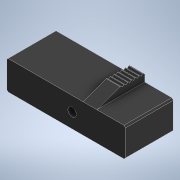
# Autodesk Inventor part: Magazin2_Stössel
Saved by Autodesk Inventor 2021 (Build 250183000, 183)
## iProperties
Created: 2024-08-28
Part Number: Magazin2_Stössel
Material: Generic
Document SubType Name: Modeling
Designer: Lukas
Density: 1 g/cm^3
Appearance: Default
Author: Lukas
Autodesk Inventor part; units mm, degrees
ref_plane "YZ Plane" through (0, 0, 0) normal (1, 0, 0) x (0, 1, 0)
ref_plane "XZ Plane" through (0, 0, 0) normal (0, 1, 0) x (-1, 0, 0)
ref_plane "XY Plane" through (0, 0, 0) normal (0, 0, 1) x (1, 0, 0)
sketch "Sketch1" plane through (0, 0, 0) normal (0, 0, 1) x (1, 0, 0)
  line L0 (-19.85, 4.85) -> (19.85, 4.85)
  line L1 (19.85, 4.85) -> (19.85, -4.85)
  line L2 (19.85, -4.85) -> (-19.85, -4.85)
  line L3 (-19.85, -4.85) -> (-19.85, 4.85)
  line L4 (5.7, 4.85) -> (5.7, 7.65)
  line L5 (5.7, 7.65) -> (10.3, 7.65)
  line L6 (10.3, 7.65) -> (10.3, 4.85)
  point P0 (0, 0)
  point P1 (0, 4.85)
  point P2 (-19.85, 0)
  point P3 (8, 7.65)
  dimension "d0" = 9.7
  dimension "d1" = 39.7
  dimension "d2" = 4.6
  dimension "d3" = 2.8
  dimension "d28" = 8
  constraints: 14 end point, 3 midpoint, 3 perpendicular, 2 parallel, 2 point on line, 1 horizontal, 1 horizontal alignment, 1 vertical, 1 vertical alignment
  measures "d0" distance of L2.end L0.start
  measures "d1" distance of L0.start L0.end
  measures "d2" distance of L4.end L5.end
  measures "d3" distance of L5.end L6.end
  measures "d28" horizontal distance of point (8, 7.65) point (0, 4.85)
extrude "Extrusion1" add sketch "Sketch1" along normal blind 16
sketch "Sketch2" plane through (10.3, 4.85, 0) normal (1, 0, 0) x (0, 0, -1)
  line L0 (0, 0) -> (0, 2.8) projected
  line L1 (0, 2.8) -> (-16, 2.8) projected
  line L2 (-16, 0) -> (-16, 2.8) projected
  line L3 (0, 0) -> (-16, 0) projected
  line L4 (0, 0) -> (-16, 0) projected
  line L5 (-16, 0) -> (-8.25, 2.8)
  line L6 (0, 2.8) -> (-16, 2.8) projected
  line L7 (-6.75, 2.8) -> (-6.25, 2.3)
  line L8 (-6.25, 2.3) -> (-5.75, 2.8)
  line L9 (-4.25, 2.8) -> (-3.75, 2.3)
  line L10 (-3.75, 2.3) -> (-3.25, 2.8)
  line L11 (-1.75, 2.8) -> (-1.25, 2.3)
  line L12 (-1.25, 2.3) -> (-0.75, 2.8)
  line L13 (0, 2.8) -> (-16, 2.8) projected
  line L14 (-3, 2.8) -> (-2.5, 2.3)
  line L15 (-2.5, 2.3) -> (-2, 2.8)
  line L16 (-5.5, 2.8) -> (-5, 2.3)
  line L17 (-5, 2.3) -> (-4.5, 2.8)
  line L18 (-7, 2.8) -> (-7.5, 2.3)
  line L19 (-7.5, 2.3) -> (-8, 2.8)
  line L20 (-0.5, 2.8) -> (0, 2.3)
  line L21 (0, 0) -> (0, 2.8) projected
  point P0 (0, -4.85)
  dimension "d8" = 0.75
  dimension "d9" = 1
  dimension "d13" = 0.25
  dimension "d14" = 0.25
  dimension "d15" = 0.25
  dimension "d16" = 0.25
  dimension "d17" = 0.25
  dimension "d18" = 0.25
  dimension "d26" = 0.5
  constraints: 28 end point, 14 perpendicular, 4 point on line, 2 horizontal alignment, 2 parallel, 14 other
  measures "d8" distance from line of L0 L12.end
  measures "d9" distance of L11.start L12.end
  measures "d13" distance of L11.start L15.end
  measures "d14" distance of L10.end L14.start
  measures "d15" distance of L17.end L9.start
  measures "d16" distance of L8.end L16.start
  measures "d17" distance of L7.start L18.start
  measures "d18" distance of L5.end L19.end
  measures "d26" distance of L0.end L20.start
extrude "Extrusion2" cut sketch "Sketch2" against normal through all contours L20 L1 L0 | L2 L1 L5 | L12 L11 L1 | L1 L18 L19 | L15 L14 L1 | L1 L8 L7 | L10 L9 L1 | L1 L17 L16
sketch "Sketch3" plane through (0, 0, 16) normal (0, 0, 1) x (1, 0, 0)
  circle A0 centre (2, 0) radius 1.4
  point P0 (0, 0)
  dimension "d19" = 2
  dimension "d20" = 2.8
  constraints: 1 centre point, 1 horizontal alignment
  measures "d19" distance of point (0, 0) A0.centre
  measures "d20" diameter of A0
extrude "Extrusion3" cut sketch "Sketch3" against normal blind 10
chamfer "Chamfer1" distance 0.5 angle 45 4 edges at (-19.85, -4.85, 8) (-19.85, 4.85, 8) (19.85, -4.85, 8) (19.85, 4.85, 8)
equation "\"d14\" = d13"
equation "\"d15\" = d14"
equation "\"d16\" = d15"
equation "\"d17\" = d16"
equation "\"d18\" = d17"
body "Solid1"
